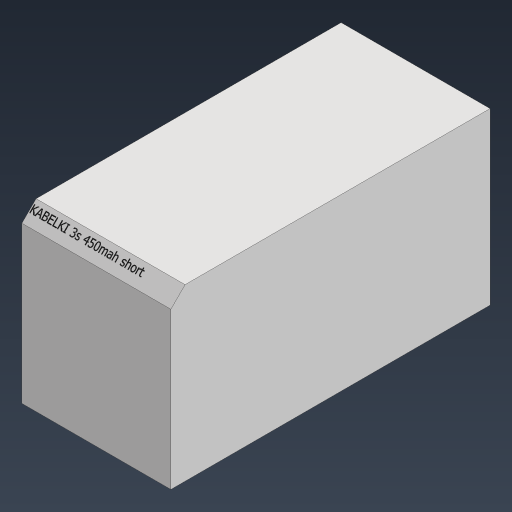
# Autodesk Inventor part: 2s450mah
Saved by Autodesk Inventor 2023 (Build 270158000, 158)
## iProperties
Created: 2026-03-09
Part Number: 2s450mah
Material: Generic
Document SubType Name: Modeling
Designer: szymo
Density: 1 g/cm^3
Appearance: Default
Author: szymo
Autodesk Inventor part; units mm, degrees
ref_plane "YZ Plane" through (0, 0, 0) normal (1, 0, 0) x (0, 1, 0)
ref_plane "XZ Plane" through (0, 0, 0) normal (0, 1, 0) x (-1, 0, 0)
ref_plane "XY Plane" through (0, 0, 0) normal (0, 0, 1) x (1, 0, 0)
sketch "Sketch1" plane through (0, 0, 0) normal (0, 1, 0) x (-1, 0, 0)
  line L0 (0, 0) -> (-21, 0)
  line L1 (-21, 0) -> (-21, -45)
  line L2 (-21, -45) -> (0, -45)
  line L3 (0, -45) -> (0, 0)
  dimension "d0" = 21
  dimension "d1" = 45
  constraints: 8 end point, 2 parallel, 1 horizontal, 1 perpendicular
  measures "d0" distance of L2.end L1.end
  measures "d1" distance of L0.end L1.end
extrude "Extrusion1" add sketch "Sketch1" along normal blind 24
chamfer "Chamfer1" distance 2 angle 45 1 edges at (10.5, 24, 0)
sketch "Sketch2" plane through (0, 24, -2) normal (0, 0.7071, 0.7071) x (1, 0, 0)
  line L0 (0.0469, -0.5129) -> (26.4473, -0.5129) construction
  line L1 (26.4473, -0.5129) -> (26.4473, -3.2591) construction
  line L2 (26.4473, -3.2591) -> (0.0469, -3.2591) construction
  line L3 (0.0469, -3.2591) -> (0.0469, -0.5129) construction
  line L4 (0.8775, -1.5575) -> (0.7049, -1.5575)
  line L5 (0.7049, -1.5575) -> (0.3395, -1.0923)
  line L6 (0.3395, -1.0923) -> (0.2811, -1.158)
  line L7 (0.2811, -1.158) -> (0.2811, -1.5575)
  line L8 (0.2811, -1.5575) -> (0.1482, -1.5575)
  line L9 (0.1482, -1.5575) -> (0.1482, -0.5575)
  line L10 (0.1482, -0.5575) -> (0.2811, -0.5575)
  line L11 (0.2811, -0.5575) -> (0.2811, -1.017)
  line L12 (0.2811, -1.017) -> (0.6912, -0.5575)
  line L13 (0.6912, -0.5575) -> (0.8532, -0.5575)
  line L14 (0.8532, -0.5575) -> (0.4391, -1.004)
  line L15 (0.4391, -1.004) -> (0.8775, -1.5575)
  line L16 (0.8492, -1.5575) -> (1.1863, -0.5575)
  line L17 (1.1863, -0.5575) -> (1.35, -0.5575)
  line L18 (1.35, -0.5575) -> (1.6871, -1.5575)
  line L19 (1.6871, -1.5575) -> (1.5469, -1.5575)
  line L20 (1.5469, -1.5575) -> (1.4561, -1.2779)
  line L21 (1.4561, -1.2779) -> (1.0745, -1.2779)
  line L22 (1.0745, -1.2779) -> (0.9837, -1.5575)
  line L23 (0.9837, -1.5575) -> (0.8492, -1.5575)
  line L24 (1.4197, -1.1644) -> (1.2649, -0.6936)
  line L25 (1.2649, -0.6936) -> (1.1109, -1.1644)
  line L26 (1.1109, -1.1644) -> (1.4197, -1.1644)
  spline S0 degree 2 poles (2.4602, -1.2503) (2.4602, -1.3249) (2.4035, -1.4392) (2.3565, -1.4764) knots 0 0 0 1 2 2 2
  spline S1 degree 2 poles (2.3565, -1.4764) (2.2997, -1.5202) (2.1709, -1.5575) (2.0688, -1.5575) knots 0 0 0 1 2 2 2
  line L27 (2.0688, -1.5575) -> (1.7819, -1.5575)
  line L28 (1.7819, -1.5575) -> (1.7819, -0.5575)
  line L29 (1.7819, -0.5575) -> (2.0469, -0.5575)
  spline S2 degree 2 poles (2.0469, -0.5575) (2.1539, -0.5575) (2.2608, -0.5713) (2.3095, -0.598) knots 0 0 0 1 2 2 2
  spline S3 degree 2 poles (2.3095, -0.598) (2.3638, -0.6264) (2.4132, -0.7196) (2.4132, -0.7828) knots 0 0 0 1 2 2 2
  spline S4 degree 2 poles (2.4132, -0.7828) (2.4132, -0.8533) (2.3386, -0.9651) (2.273, -0.9967) knots 0 0 0 1 2 2 2
  line L30 (2.273, -0.9967) -> (2.273, -1.0016)
  spline S5 degree 2 poles (2.273, -1.0016) (2.3621, -1.0259) (2.4602, -1.1547) (2.4602, -1.2503) knots 0 0 0 1 2 2 2
  spline S6 degree 2 poles (2.3216, -1.256) (2.3216, -1.1993) (2.2892, -1.1264) (2.2406, -1.1004) knots 0 0 0 1 2 2 2
  spline S7 degree 2 poles (2.2406, -1.1004) (2.209, -1.0842) (2.1344, -1.0745) (2.0655, -1.0745) knots 0 0 0 1 2 2 2
  line L31 (2.0655, -1.0745) -> (1.9148, -1.0745)
  line L32 (1.9148, -1.0745) -> (1.9148, -1.444)
  line L33 (1.9148, -1.444) -> (2.0226, -1.444)
  spline S8 degree 2 poles (2.0226, -1.444) (2.1101, -1.444) (2.2106, -1.4278) (2.2495, -1.4019) knots 0 0 0 1 2 2 2
  spline S9 degree 2 poles (2.2495, -1.4019) (2.2868, -1.3751) (2.3216, -1.3087) (2.3216, -1.256) knots 0 0 0 1 2 2 2
  spline S10 degree 2 poles (2.2746, -0.8014) (2.2746, -0.7657) (2.2503, -0.7123) (2.2236, -0.6969) knots 0 0 0 1 2 2 2
  spline S11 degree 2 poles (2.2236, -0.6969) (2.1912, -0.679) (2.1125, -0.6709) (2.042, -0.6709) knots 0 0 0 1 2 2 2
  line L34 (2.042, -0.6709) -> (1.9148, -0.6709)
  line L35 (1.9148, -0.6709) -> (1.9148, -0.9635)
  line L36 (1.9148, -0.9635) -> (2.0655, -0.9635)
  spline S12 degree 2 poles (2.0655, -0.9635) (2.1279, -0.9635) (2.1871, -0.9505) (2.2187, -0.9303) knots 0 0 0 1 2 2 2
  spline S13 degree 2 poles (2.2187, -0.9303) (2.2495, -0.9108) (2.2746, -0.8484) (2.2746, -0.8014) knots 0 0 0 1 2 2 2
  line L37 (2.5923, -1.5575) -> (2.5923, -0.5575)
  line L38 (2.5923, -0.5575) -> (3.2179, -0.5575)
  line L39 (3.2179, -0.5575) -> (3.2179, -0.6758)
  line L40 (3.2179, -0.6758) -> (2.7252, -0.6758)
  line L41 (2.7252, -0.6758) -> (2.7252, -0.9497)
  line L42 (2.7252, -0.9497) -> (3.1847, -0.9497)
  line L43 (3.1847, -0.9497) -> (3.1847, -1.068)
  line L44 (3.1847, -1.068) -> (2.7252, -1.068)
  line L45 (2.7252, -1.068) -> (2.7252, -1.4392)
  line L46 (2.7252, -1.4392) -> (3.2179, -1.4392)
  line L47 (3.2179, -1.4392) -> (3.2179, -1.5575)
  line L48 (3.2179, -1.5575) -> (2.5923, -1.5575)
  line L49 (3.9432, -1.5575) -> (3.3638, -1.5575)
  line L50 (3.3638, -1.5575) -> (3.3638, -0.5575)
  line L51 (3.3638, -0.5575) -> (3.4967, -0.5575)
  line L52 (3.4967, -0.5575) -> (3.4967, -1.4392)
  line L53 (3.4967, -1.4392) -> (3.9432, -1.4392)
  line L54 (3.9432, -1.4392) -> (3.9432, -1.5575)
  line L55 (4.7771, -1.5575) -> (4.6044, -1.5575)
  line L56 (4.6044, -1.5575) -> (4.239, -1.0923)
  line L57 (4.239, -1.0923) -> (4.1806, -1.158)
  line L58 (4.1806, -1.158) -> (4.1806, -1.5575)
  line L59 (4.1806, -1.5575) -> (4.0477, -1.5575)
  line L60 (4.0477, -1.5575) -> (4.0477, -0.5575)
  line L61 (4.0477, -0.5575) -> (4.1806, -0.5575)
  line L62 (4.1806, -0.5575) -> (4.1806, -1.017)
  line L63 (4.1806, -1.017) -> (4.5907, -0.5575)
  line L64 (4.5907, -0.5575) -> (4.7527, -0.5575)
  line L65 (4.7527, -0.5575) -> (4.3386, -1.004)
  line L66 (4.3386, -1.004) -> (4.7771, -1.5575)
  line L67 (5.2049, -1.5575) -> (4.8176, -1.5575)
  line L68 (4.8176, -1.5575) -> (4.8176, -1.4554)
  line L69 (4.8176, -1.4554) -> (4.9448, -1.4554)
  line L70 (4.9448, -1.4554) -> (4.9448, -0.6596)
  line L71 (4.9448, -0.6596) -> (4.8176, -0.6596)
  line L72 (4.8176, -0.6596) -> (4.8176, -0.5575)
  line L73 (4.8176, -0.5575) -> (5.2049, -0.5575)
  line L74 (5.2049, -0.5575) -> (5.2049, -0.6596)
  line L75 (5.2049, -0.6596) -> (5.0777, -0.6596)
  line L76 (5.0777, -0.6596) -> (5.0777, -1.4554)
  line L77 (5.0777, -1.4554) -> (5.2049, -1.4554)
  line L78 (5.2049, -1.4554) -> (5.2049, -1.5575)
  spline S14 degree 2 poles (6.0404, -0.6523) (6.004, -0.6523) (5.9318, -0.6701) (5.897, -0.6839) knots 0 0 0 1 2 2 2
  spline S15 degree 2 poles (5.897, -0.6839) (5.8646, -0.6977) (5.8168, -0.7268) (5.7981, -0.7398) knots 0 0 0 1 2 2 2
  line L79 (5.7981, -0.7398) -> (5.79, -0.7398)
  line L80 (5.79, -0.7398) -> (5.79, -0.598)
  spline S16 degree 2 poles (5.79, -0.598) (5.8338, -0.5745) (5.9837, -0.5364) (6.051, -0.5364) knots 0 0 0 1 2 2 2
  spline S17 degree 2 poles (6.051, -0.5364) (6.119, -0.5364) (6.2203, -0.564) (6.2617, -0.5931) knots 0 0 0 1 2 2 2
  spline S18 degree 2 poles (6.2617, -0.5931) (6.3054, -0.6247) (6.3508, -0.7163) (6.3508, -0.7779) knots 0 0 0 1 2 2 2
  spline S19 degree 2 poles (6.3508, -0.7779) (6.3508, -0.8606) (6.2422, -0.9854) (6.166, -1.0016) knots 0 0 0 1 2 2 2
  line L81 (6.166, -1.0016) -> (6.166, -1.0113)
  spline S20 degree 2 poles (6.166, -1.0113) (6.1976, -1.0178) (6.2698, -1.0469) (6.3006, -1.0761) knots 0 0 0 1 2 2 2
  spline S21 degree 2 poles (6.3006, -1.0761) (6.3313, -1.1045) (6.3702, -1.1952) (6.3702, -1.2609) knots 0 0 0 1 2 2 2
  spline S22 degree 2 poles (6.3702, -1.2609) (6.3702, -1.3281) (6.3241, -1.4424) (6.2819, -1.4862) knots 0 0 0 1 2 2 2
  spline S23 degree 2 poles (6.2819, -1.4862) (6.2382, -1.5315) (6.1142, -1.5785) (6.0356, -1.5785) knots 0 0 0 1 2 2 2
  spline S24 degree 2 poles (6.0356, -1.5785) (5.9602, -1.5785) (5.8127, -1.5421) (5.7625, -1.517) knots 0 0 0 1 2 2 2
  line L82 (5.7625, -1.517) -> (5.7625, -1.3751)
  line L83 (5.7625, -1.3751) -> (5.7722, -1.3751)
  spline S25 degree 2 poles (5.7722, -1.3751) (5.8143, -1.4059) (5.957, -1.4627) (6.0275, -1.4627) knots 0 0 0 1 2 2 2
  spline S26 degree 2 poles (6.0275, -1.4627) (6.0688, -1.4627) (6.1514, -1.4367) (6.179, -1.4067) knots 0 0 0 1 2 2 2
  spline S27 degree 2 poles (6.179, -1.4067) (6.2057, -1.3768) (6.2341, -1.3055) (6.2341, -1.2512) knots 0 0 0 1 2 2 2
  spline S28 degree 2 poles (6.2341, -1.2512) (6.2341, -1.1969) (6.2025, -1.1264) (6.1741, -1.1061) knots 0 0 0 1 2 2 2
  spline S29 degree 2 poles (6.1741, -1.1061) (6.1458, -1.0858) (6.0688, -1.0704) (6.0234, -1.0704) knots 0 0 0 1 2 2 2
  line L84 (6.0234, -1.0704) -> (5.9667, -1.0704)
  line L85 (5.9667, -1.0704) -> (5.9667, -0.9594)
  line L86 (5.9667, -0.9594) -> (6.0113, -0.9594)
  spline S30 degree 2 poles (6.0113, -0.9594) (6.1012, -0.9594) (6.2147, -0.8735) (6.2147, -0.7917) knots 0 0 0 1 2 2 2
  spline S31 degree 2 poles (6.2147, -0.7917) (6.2147, -0.7536) (6.1855, -0.6993) (6.162, -0.6831) knots 0 0 0 1 2 2 2
  spline S32 degree 2 poles (6.162, -0.6831) (6.1369, -0.6661) (6.0753, -0.6523) (6.0404, -0.6523) knots 0 0 0 1 2 2 2
  spline S33 degree 2 poles (6.7422, -1.5753) (6.6668, -1.5753) (6.5364, -1.5348) (6.4934, -1.5121) knots 0 0 0 1 2 2 2
  line L87 (6.4934, -1.5121) -> (6.4934, -1.3703)
  line L88 (6.4934, -1.3703) -> (6.4999, -1.3703)
  spline S34 degree 2 poles (6.4999, -1.3703) (6.5161, -1.3832) (6.5599, -1.414) (6.5963, -1.4311) knots 0 0 0 1 2 2 2
  spline S35 degree 2 poles (6.5963, -1.4311) (6.6279, -1.4465) (6.7057, -1.4691) (6.7471, -1.4691) knots 0 0 0 1 2 2 2
  spline S36 degree 2 poles (6.7471, -1.4691) (6.7771, -1.4691) (6.8459, -1.4554) (6.8621, -1.444) knots 0 0 0 1 2 2 2
  spline S37 degree 2 poles (6.8621, -1.444) (6.8856, -1.4286) (6.9067, -1.3938) (6.9067, -1.3581) knots 0 0 0 1 2 2 2
  spline S38 degree 2 poles (6.9067, -1.3581) (6.9067, -1.3136) (6.8581, -1.2674) (6.7957, -1.252) knots 0 0 0 1 2 2 2
  spline S39 degree 2 poles (6.7957, -1.252) (6.7714, -1.2463) (6.6936, -1.2301) (6.6604, -1.2212) knots 0 0 0 1 2 2 2
  spline S40 degree 2 poles (6.6604, -1.2212) (6.5745, -1.1961) (6.4967, -1.0923) (6.4967, -1.0186) knots 0 0 0 1 2 2 2
  spline S41 degree 2 poles (6.4967, -1.0186) (6.4967, -0.9165) (6.6498, -0.7892) (6.7762, -0.7892) knots 0 0 0 1 2 2 2
  spline S42 degree 2 poles (6.7762, -0.7892) (6.8386, -0.7892) (6.9651, -0.82) (7.008, -0.8435) knots 0 0 0 1 2 2 2
  line L89 (7.008, -0.8435) -> (7.008, -0.9789)
  line L90 (7.008, -0.9789) -> (7.0015, -0.9789)
  spline S43 degree 2 poles (7.0015, -0.9789) (6.9529, -0.94) (6.8346, -0.8954) (6.7738, -0.8954) knots 0 0 0 1 2 2 2
  spline S44 degree 2 poles (6.7738, -0.8954) (6.7114, -0.8954) (6.6255, -0.9481) (6.6255, -1.0008) knots 0 0 0 1 2 2 2
  spline S45 degree 2 poles (6.6255, -1.0008) (6.6255, -1.0486) (6.6766, -1.0948) (6.7333, -1.1093) knots 0 0 0 1 2 2 2
  spline S46 degree 2 poles (6.7333, -1.1093) (6.7608, -1.1166) (6.8305, -1.1312) (6.8686, -1.1401) knots 0 0 0 1 2 2 2
  spline S47 degree 2 poles (6.8686, -1.1401) (6.9513, -1.1612) (7.0356, -1.2576) (7.0356, -1.3411) knots 0 0 0 1 2 2 2
  spline S48 degree 2 poles (7.0356, -1.3411) (7.0356, -1.3897) (6.9975, -1.4756) (6.9602, -1.5072) knots 0 0 0 1 2 2 2
  spline S49 degree 2 poles (6.9602, -1.5072) (6.9205, -1.5405) (6.8192, -1.5753) (6.7422, -1.5753) knots 0 0 0 1 2 2 2
  line L91 (8.2074, -1.2139) -> (8.0882, -1.2139)
  line L92 (8.0882, -1.2139) -> (8.0882, -1.5575)
  line L93 (8.0882, -1.5575) -> (7.9594, -1.5575)
  line L94 (7.9594, -1.5575) -> (7.9594, -1.2139)
  line L95 (7.9594, -1.2139) -> (7.5177, -1.2139)
  line L96 (7.5177, -1.2139) -> (7.5177, -1.0729)
  line L97 (7.5177, -1.0729) -> (7.9651, -0.5575)
  line L98 (7.9651, -0.5575) -> (8.0882, -0.5575)
  line L99 (8.0882, -0.5575) -> (8.0882, -1.1061)
  line L100 (8.0882, -1.1061) -> (8.2074, -1.1061)
  line L101 (8.2074, -1.1061) -> (8.2074, -1.2139)
  line L102 (7.9594, -1.1061) -> (7.9594, -0.7155)
  line L103 (7.9594, -0.7155) -> (7.6231, -1.1061)
  line L104 (7.6231, -1.1061) -> (7.9594, -1.1061)
  spline S50 degree 2 poles (8.9205, -1.2398) (8.9205, -1.3119) (8.8743, -1.4351) (8.8322, -1.4805) knots 0 0 0 1 2 2 2
  spline S51 degree 2 poles (8.8322, -1.4805) (8.79, -1.5259) (8.6644, -1.5785) (8.5866, -1.5785) knots 0 0 0 1 2 2 2
  spline S52 degree 2 poles (8.5866, -1.5785) (8.5153, -1.5785) (8.3759, -1.5469) (8.3249, -1.5218) knots 0 0 0 1 2 2 2
  line L105 (8.3249, -1.5218) -> (8.3249, -1.38)
  line L106 (8.3249, -1.38) -> (8.3346, -1.38)
  spline S53 degree 2 poles (8.3346, -1.38) (8.35, -1.3914) (8.4075, -1.4205) (8.4424, -1.4335) knots 0 0 0 1 2 2 2
  spline S54 degree 2 poles (8.4424, -1.4335) (8.4821, -1.4473) (8.5477, -1.4627) (8.589, -1.4627) knots 0 0 0 1 2 2 2
  spline S55 degree 2 poles (8.589, -1.4627) (8.6296, -1.4627) (8.7057, -1.4335) (8.7333, -1.4019) knots 0 0 0 1 2 2 2
  spline S56 degree 2 poles (8.7333, -1.4019) (8.7584, -1.3719) (8.7843, -1.2925) (8.7843, -1.239) knots 0 0 0 1 2 2 2
  spline S57 degree 2 poles (8.7843, -1.239) (8.7843, -1.1855) (8.7552, -1.1174) (8.7276, -1.0948) knots 0 0 0 1 2 2 2
  spline S58 degree 2 poles (8.7276, -1.0948) (8.6993, -1.0696) (8.615, -1.0486) (8.5639, -1.0486) knots 0 0 0 1 2 2 2
  spline S59 degree 2 poles (8.5639, -1.0486) (8.5088, -1.0486) (8.3994, -1.0656) (8.3662, -1.0729) knots 0 0 0 1 2 2 2
  line L107 (8.3662, -1.0729) -> (8.3662, -0.5575)
  line L108 (8.3662, -0.5575) -> (8.9148, -0.5575)
  line L109 (8.9148, -0.5575) -> (8.9148, -0.675)
  line L110 (8.9148, -0.675) -> (8.495, -0.675)
  line L111 (8.495, -0.675) -> (8.495, -0.9416)
  spline S60 degree 2 poles (8.495, -0.9416) (8.5194, -0.9384) (8.5664, -0.9359) (8.5858, -0.9359) knots 0 0 0 1 2 2 2
  spline S61 degree 2 poles (8.5858, -0.9359) (8.6628, -0.9359) (8.7689, -0.961) (8.8176, -0.9983) knots 0 0 0 1 2 2 2
  spline S62 degree 2 poles (8.8176, -0.9983) (8.867, -1.0356) (8.9205, -1.1491) (8.9205, -1.2398) knots 0 0 0 1 2 2 2
  spline S63 degree 2 poles (9.6871, -1.0575) (9.6871, -1.3265) (9.5307, -1.5785) (9.3678, -1.5785) knots 0 0 0 1 2 2 2
  spline S64 degree 2 poles (9.3678, -1.5785) (9.2025, -1.5785) (9.0477, -1.3217) (9.0477, -1.0583) knots 0 0 0 1 2 2 2
  spline S65 degree 2 poles (9.0477, -1.0583) (9.0477, -0.7876) (9.2041, -0.5372) (9.3678, -0.5372) knots 0 0 0 1 2 2 2
  spline S66 degree 2 poles (9.3678, -0.5372) (9.5323, -0.5372) (9.6871, -0.7965) (9.6871, -1.0575) knots 0 0 0 1 2 2 2
  spline S67 degree 2 poles (9.5153, -1.3622) (9.5348, -1.3127) (9.551, -1.1604) (9.551, -1.0575) knots 0 0 0 1 2 2 2
  spline S68 degree 2 poles (9.551, -1.0575) (9.551, -0.9546) (9.5348, -0.803) (9.5145, -0.752) knots 0 0 0 1 2 2 2
  spline S69 degree 2 poles (9.5145, -0.752) (9.4942, -0.7009) (9.4237, -0.6482) (9.3678, -0.6482) knots 0 0 0 1 2 2 2
  spline S70 degree 2 poles (9.3678, -0.6482) (9.3119, -0.6482) (9.2398, -0.7009) (9.2187, -0.7536) knots 0 0 0 1 2 2 2
  spline S71 degree 2 poles (9.2187, -0.7536) (9.1984, -0.8046) (9.1839, -0.9602) (9.1839, -1.0583) knots 0 0 0 1 2 2 2
  spline S72 degree 2 poles (9.1839, -1.0583) (9.1839, -1.1636) (9.1968, -1.3046) (9.2179, -1.3597) knots 0 0 0 1 2 2 2
  spline S73 degree 2 poles (9.2179, -1.3597) (9.2373, -1.4116) (9.3095, -1.4675) (9.3678, -1.4675) knots 0 0 0 1 2 2 2
  spline S74 degree 2 poles (9.3678, -1.4675) (9.4229, -1.4675) (9.495, -1.4149) (9.5153, -1.3622) knots 0 0 0 1 2 2 2
  line L112 (10.6847, -1.5575) -> (10.6847, -1.1231)
  spline S75 degree 2 poles (10.6847, -1.1231) (10.6847, -1.0713) (10.6766, -0.9829) (10.6636, -0.9586) knots 0 0 0 1 2 2 2
  spline S76 degree 2 poles (10.6636, -0.9586) (10.6506, -0.9319) (10.6012, -0.9059) (10.5583, -0.9059) knots 0 0 0 1 2 2 2
  spline S77 degree 2 poles (10.5583, -0.9059) (10.5194, -0.9059) (10.4302, -0.9538) (10.3832, -0.9991) knots 0 0 0 1 2 2 2
  spline S78 degree 2 poles (10.3832, -0.9991) (10.384, -1.0105) (10.3856, -1.0421) (10.3856, -1.0632) knots 0 0 0 1 2 2 2
  line L113 (10.3856, -1.0632) -> (10.3856, -1.5575)
  line L114 (10.3856, -1.5575) -> (10.2592, -1.5575)
  line L115 (10.2592, -1.5575) -> (10.2592, -1.1231)
  spline S79 degree 2 poles (10.2592, -1.1231) (10.2592, -1.0713) (10.2511, -0.9829) (10.2382, -0.9586) knots 0 0 0 1 2 2 2
  spline S80 degree 2 poles (10.2382, -0.9586) (10.2252, -0.9319) (10.1758, -0.9059) (10.1328, -0.9059) knots 0 0 0 1 2 2 2
  spline S81 degree 2 poles (10.1328, -0.9059) (10.0923, -0.9059) (10.0023, -0.957) (9.9602, -0.9967) knots 0 0 0 1 2 2 2
  line L116 (9.9602, -0.9967) -> (9.9602, -1.5575)
  line L117 (9.9602, -1.5575) -> (9.8338, -1.5575)
  line L118 (9.8338, -1.5575) -> (9.8338, -0.8071)
  line L119 (9.8338, -0.8071) -> (9.9602, -0.8071)
  line L120 (9.9602, -0.8071) -> (9.9602, -0.8897)
  spline S82 degree 2 poles (9.9602, -0.8897) (10.0096, -0.8403) (10.1069, -0.786) (10.1652, -0.786) knots 0 0 0 1 2 2 2
  spline S83 degree 2 poles (10.1652, -0.786) (10.2317, -0.786) (10.3346, -0.8468) (10.3613, -0.9157) knots 0 0 0 1 2 2 2
  spline S84 degree 2 poles (10.3613, -0.9157) (10.4189, -0.8516) (10.5275, -0.786) (10.5907, -0.786) knots 0 0 0 1 2 2 2
  spline S85 degree 2 poles (10.5907, -0.786) (10.6393, -0.786) (10.7187, -0.816) (10.7479, -0.85) knots 0 0 0 1 2 2 2
  spline S86 degree 2 poles (10.7479, -0.85) (10.7779, -0.8841) (10.8111, -0.9862) (10.8111, -1.0632) knots 0 0 0 1 2 2 2
  line L121 (10.8111, -1.0632) -> (10.8111, -1.5575)
  line L122 (10.8111, -1.5575) -> (10.6847, -1.5575)
  spline S87 degree 2 poles (11.4067, -1.4781) (11.3913, -1.4894) (11.3395, -1.5299) (11.3151, -1.5421) knots 0 0 0 1 2 2 2
  spline S88 degree 2 poles (11.3151, -1.5421) (11.2819, -1.5599) (11.2195, -1.5785) (11.1628, -1.5785) knots 0 0 0 1 2 2 2
  spline S89 degree 2 poles (11.1628, -1.5785) (11.1166, -1.5785) (11.0331, -1.5437) (11.0015, -1.5121) knots 0 0 0 1 2 2 2
  spline S90 degree 2 poles (11.0015, -1.5121) (10.9715, -1.4813) (10.9351, -1.3905) (10.9351, -1.3403) knots 0 0 0 1 2 2 2
  spline S91 degree 2 poles (10.9351, -1.3403) (10.9351, -1.2625) (11.0007, -1.1523) (11.072, -1.1207) knots 0 0 0 1 2 2 2
  spline S92 degree 2 poles (11.072, -1.1207) (11.1352, -1.0915) (11.307, -1.0696) (11.4067, -1.064) knots 0 0 0 1 2 2 2
  line L123 (11.4067, -1.064) -> (11.4067, -1.0397)
  spline S93 degree 2 poles (11.4067, -1.0397) (11.4067, -0.9959) (11.38, -0.9416) (11.3557, -0.9262) knots 0 0 0 1 2 2 2
  spline S94 degree 2 poles (11.3557, -0.9262) (11.3313, -0.9108) (11.2617, -0.9011) (11.2244, -0.9011) knots 0 0 0 1 2 2 2
  spline S95 degree 2 poles (11.2244, -0.9011) (11.1806, -0.9011) (11.0623, -0.927) (11.0031, -0.9521) knots 0 0 0 1 2 2 2
  line L124 (11.0031, -0.9521) -> (10.9959, -0.9521)
  line L125 (10.9959, -0.9521) -> (10.9959, -0.8233)
  spline S96 degree 2 poles (10.9959, -0.8233) (11.0307, -0.8136) (11.1612, -0.7892) (11.2252, -0.7892) knots 0 0 0 1 2 2 2
  spline S97 degree 2 poles (11.2252, -0.7892) (11.303, -0.7892) (11.4091, -0.8136) (11.4513, -0.8452) knots 0 0 0 1 2 2 2
  spline S98 degree 2 poles (11.4513, -0.8452) (11.4926, -0.876) (11.5331, -0.974) (11.5331, -1.0445) knots 0 0 0 1 2 2 2
  line L126 (11.5331, -1.0445) -> (11.5331, -1.5575)
  line L127 (11.5331, -1.5575) -> (11.4067, -1.5575)
  line L128 (11.4067, -1.5575) -> (11.4067, -1.4781)
  line L129 (11.4067, -1.3727) -> (11.4067, -1.1644)
  spline S99 degree 2 poles (11.4067, -1.1644) (11.3613, -1.1685) (11.2244, -1.1823) (11.1814, -1.1952) knots 0 0 0 1 2 2 2
  spline S100 degree 2 poles (11.1814, -1.1952) (11.1312, -1.2106) (11.0655, -1.2747) (11.0655, -1.3314) knots 0 0 0 1 2 2 2
  spline S101 degree 2 poles (11.0655, -1.3314) (11.0655, -1.3962) (11.1385, -1.4619) (11.2082, -1.4619) knots 0 0 0 1 2 2 2
  spline S102 degree 2 poles (11.2082, -1.4619) (11.2673, -1.4619) (11.3646, -1.4108) (11.4067, -1.3727) knots 0 0 0 1 2 2 2
  line L130 (12.2997, -1.5575) -> (12.1733, -1.5575)
  line L131 (12.1733, -1.5575) -> (12.1733, -1.1296)
  spline S103 degree 2 poles (12.1733, -1.1296) (12.1733, -1.0777) (12.1636, -0.9886) (12.149, -0.9619) knots 0 0 0 1 2 2 2
  spline S104 degree 2 poles (12.149, -0.9619) (12.1336, -0.9335) (12.0785, -0.9059) (12.0315, -0.9059) knots 0 0 0 1 2 2 2
  spline S105 degree 2 poles (12.0315, -0.9059) (11.9845, -0.9059) (11.8848, -0.9562) (11.837, -0.9967) knots 0 0 0 1 2 2 2
  line L132 (11.837, -0.9967) -> (11.837, -1.5575)
  line L133 (11.837, -1.5575) -> (11.7106, -1.5575)
  line L134 (11.7106, -1.5575) -> (11.7106, -0.5129)
  line L135 (11.7106, -0.5129) -> (11.837, -0.5129)
  line L136 (11.837, -0.5129) -> (11.837, -0.8905)
  spline S106 degree 2 poles (11.837, -0.8905) (11.8937, -0.8395) (12.0031, -0.786) (12.0647, -0.786) knots 0 0 0 1 2 2 2
  spline S107 degree 2 poles (12.0647, -0.786) (12.1749, -0.786) (12.2997, -0.9319) (12.2997, -1.0704) knots 0 0 0 1 2 2 2
  line L137 (12.2997, -1.0704) -> (12.2997, -1.5575)
  spline S108 degree 2 poles (13.1093, -1.5753) (13.0339, -1.5753) (12.9035, -1.5348) (12.8605, -1.5121) knots 0 0 0 1 2 2 2
  line L138 (12.8605, -1.5121) -> (12.8605, -1.3703)
  line L139 (12.8605, -1.3703) -> (12.867, -1.3703)
  spline S109 degree 2 poles (12.867, -1.3703) (12.8832, -1.3832) (12.927, -1.414) (12.9634, -1.4311) knots 0 0 0 1 2 2 2
  spline S110 degree 2 poles (12.9634, -1.4311) (12.995, -1.4465) (13.0728, -1.4691) (13.1142, -1.4691) knots 0 0 0 1 2 2 2
  spline S111 degree 2 poles (13.1142, -1.4691) (13.1442, -1.4691) (13.213, -1.4554) (13.2292, -1.444) knots 0 0 0 1 2 2 2
  spline S112 degree 2 poles (13.2292, -1.444) (13.2527, -1.4286) (13.2738, -1.3938) (13.2738, -1.3581) knots 0 0 0 1 2 2 2
  spline S113 degree 2 poles (13.2738, -1.3581) (13.2738, -1.3136) (13.2252, -1.2674) (13.1628, -1.252) knots 0 0 0 1 2 2 2
  spline S114 degree 2 poles (13.1628, -1.252) (13.1385, -1.2463) (13.0607, -1.2301) (13.0275, -1.2212) knots 0 0 0 1 2 2 2
  spline S115 degree 2 poles (13.0275, -1.2212) (12.9416, -1.1961) (12.8638, -1.0923) (12.8638, -1.0186) knots 0 0 0 1 2 2 2
  spline S116 degree 2 poles (12.8638, -1.0186) (12.8638, -0.9165) (13.0169, -0.7892) (13.1433, -0.7892) knots 0 0 0 1 2 2 2
  spline S117 degree 2 poles (13.1433, -0.7892) (13.2057, -0.7892) (13.3322, -0.82) (13.3751, -0.8435) knots 0 0 0 1 2 2 2
  line L140 (13.3751, -0.8435) -> (13.3751, -0.9789)
  line L141 (13.3751, -0.9789) -> (13.3686, -0.9789)
  spline S118 degree 2 poles (13.3686, -0.9789) (13.32, -0.94) (13.2017, -0.8954) (13.1409, -0.8954) knots 0 0 0 1 2 2 2
  spline S119 degree 2 poles (13.1409, -0.8954) (13.0785, -0.8954) (12.9926, -0.9481) (12.9926, -1.0008) knots 0 0 0 1 2 2 2
  spline S120 degree 2 poles (12.9926, -1.0008) (12.9926, -1.0486) (13.0437, -1.0948) (13.1004, -1.1093) knots 0 0 0 1 2 2 2
  spline S121 degree 2 poles (13.1004, -1.1093) (13.1279, -1.1166) (13.1976, -1.1312) (13.2357, -1.1401) knots 0 0 0 1 2 2 2
  spline S122 degree 2 poles (13.2357, -1.1401) (13.3184, -1.1612) (13.4027, -1.2576) (13.4027, -1.3411) knots 0 0 0 1 2 2 2
  spline S123 degree 2 poles (13.4027, -1.3411) (13.4027, -1.3897) (13.3646, -1.4756) (13.3273, -1.5072) knots 0 0 0 1 2 2 2
  spline S124 degree 2 poles (13.3273, -1.5072) (13.2876, -1.5405) (13.1863, -1.5753) (13.1093, -1.5753) knots 0 0 0 1 2 2 2
  line L142 (14.1093, -1.5575) -> (13.9829, -1.5575)
  line L143 (13.9829, -1.5575) -> (13.9829, -1.1296)
  spline S125 degree 2 poles (13.9829, -1.1296) (13.9829, -1.0777) (13.9732, -0.9886) (13.9586, -0.9619) knots 0 0 0 1 2 2 2
  spline S126 degree 2 poles (13.9586, -0.9619) (13.9432, -0.9335) (13.8881, -0.9059) (13.8411, -0.9059) knots 0 0 0 1 2 2 2
  spline S127 degree 2 poles (13.8411, -0.9059) (13.7941, -0.9059) (13.6944, -0.9562) (13.6466, -0.9967) knots 0 0 0 1 2 2 2
  line L144 (13.6466, -0.9967) -> (13.6466, -1.5575)
  line L145 (13.6466, -1.5575) -> (13.5202, -1.5575)
  line L146 (13.5202, -1.5575) -> (13.5202, -0.5129)
  line L147 (13.5202, -0.5129) -> (13.6466, -0.5129)
  line L148 (13.6466, -0.5129) -> (13.6466, -0.8905)
  spline S128 degree 2 poles (13.6466, -0.8905) (13.7033, -0.8395) (13.8127, -0.786) (13.8743, -0.786) knots 0 0 0 1 2 2 2
  spline S129 degree 2 poles (13.8743, -0.786) (13.9845, -0.786) (14.1093, -0.9319) (14.1093, -1.0704) knots 0 0 0 1 2 2 2
  line L149 (14.1093, -1.0704) -> (14.1093, -1.5575)
  spline S130 degree 2 poles (14.9035, -1.1823) (14.9035, -1.3719) (14.7211, -1.5785) (14.5688, -1.5785) knots 0 0 0 1 2 2 2
  spline S131 degree 2 poles (14.5688, -1.5785) (14.4124, -1.5785) (14.2333, -1.3654) (14.2333, -1.1823) knots 0 0 0 1 2 2 2
  spline S132 degree 2 poles (14.2333, -1.1823) (14.2333, -0.9943) (14.4181, -0.786) (14.5688, -0.786) knots 0 0 0 1 2 2 2
  spline S133 degree 2 poles (14.5688, -0.786) (14.7211, -0.786) (14.9035, -0.9935) (14.9035, -1.1823) knots 0 0 0 1 2 2 2
  spline S134 degree 2 poles (14.773, -1.1823) (14.773, -1.0364) (14.6668, -0.8946) (14.5688, -0.8946) knots 0 0 0 1 2 2 2
  spline S135 degree 2 poles (14.5688, -0.8946) (14.4707, -0.8946) (14.3638, -1.0364) (14.3638, -1.1823) knots 0 0 0 1 2 2 2
  spline S136 degree 2 poles (14.3638, -1.1823) (14.3638, -1.3241) (14.4707, -1.47) (14.5688, -1.47) knots 0 0 0 1 2 2 2
  spline S137 degree 2 poles (14.5688, -1.47) (14.666, -1.47) (14.773, -1.3265) (14.773, -1.1823) knots 0 0 0 1 2 2 2
  line L150 (15.431, -0.9424) -> (15.4245, -0.9424)
  spline S138 degree 2 poles (15.4245, -0.9424) (15.41, -0.9384) (15.3783, -0.9367) (15.3565, -0.9367) knots 0 0 0 1 2 2 2
  spline S139 degree 2 poles (15.3565, -0.9367) (15.3054, -0.9367) (15.2049, -0.9813) (15.1595, -1.0251) knots 0 0 0 1 2 2 2
  line L151 (15.1595, -1.0251) -> (15.1595, -1.5575)
  line L152 (15.1595, -1.5575) -> (15.0331, -1.5575)
  line L153 (15.0331, -1.5575) -> (15.0331, -0.8071)
  line L154 (15.0331, -0.8071) -> (15.1595, -0.8071)
  line L155 (15.1595, -0.8071) -> (15.1595, -0.9189)
  spline S140 degree 2 poles (15.1595, -0.9189) (15.2284, -0.8573) (15.3313, -0.8071) (15.38, -0.8071) knots 0 0 0 1 2 2 2
  spline S141 degree 2 poles (15.38, -0.8071) (15.3994, -0.8071) (15.4189, -0.8087) (15.431, -0.8111) knots 0 0 0 1 2 2 2
  line L156 (15.431, -0.8111) -> (15.431, -0.9424)
  spline S142 degree 2 poles (15.756, -1.5721) (15.6531, -1.5721) (15.5372, -1.4546) (15.5372, -1.3273) knots 0 0 0 1 2 2 2
  line L157 (15.5372, -1.3273) -> (15.5372, -0.9116)
  line L158 (15.5372, -0.9116) -> (15.4521, -0.9116)
  line L159 (15.4521, -0.9116) -> (15.4521, -0.8071)
  line L160 (15.4521, -0.8071) -> (15.5372, -0.8071)
  line L161 (15.5372, -0.8071) -> (15.5372, -0.5915)
  line L162 (15.5372, -0.5915) -> (15.6636, -0.5915)
  line L163 (15.6636, -0.5915) -> (15.6636, -0.8071)
  line L164 (15.6636, -0.8071) -> (15.8962, -0.8071)
  line L165 (15.8962, -0.8071) -> (15.8962, -0.9116)
  line L166 (15.8962, -0.9116) -> (15.6636, -0.9116)
  line L167 (15.6636, -0.9116) -> (15.6636, -1.269)
  spline S143 degree 2 poles (15.6636, -1.269) (15.6636, -1.3257) (15.6677, -1.3881) (15.6814, -1.4149) knots 0 0 0 1 2 2 2
  spline S144 degree 2 poles (15.6814, -1.4149) (15.6928, -1.4384) (15.7438, -1.4619) (15.7876, -1.4619) knots 0 0 0 1 2 2 2
  spline S145 degree 2 poles (15.7876, -1.4619) (15.8184, -1.4619) (15.8759, -1.4432) (15.8889, -1.4375) knots 0 0 0 1 2 2 2
  line L168 (15.8889, -1.4375) -> (15.8962, -1.4375)
  line L169 (15.8962, -1.4375) -> (15.8962, -1.551)
  spline S146 degree 2 poles (15.8962, -1.551) (15.8605, -1.5607) (15.7876, -1.5721) (15.756, -1.5721) knots 0 0 0 1 2 2 2
  point P0 (0, -18.3848)
  constraints: 2 other
extrude "Extrusion2" cut sketch "Sketch2" against normal blind 1
body "Solid1"
